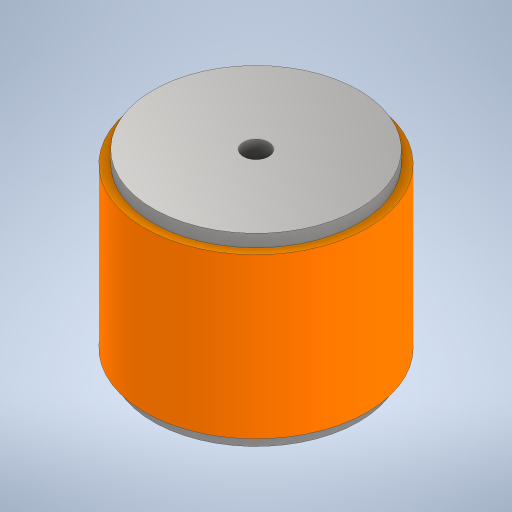
# Autodesk Inventor part: kolo
Saved by Autodesk Inventor 2024 (Build 280153000, 153)
## iProperties
Created: 2023-03-19
Part Number: kolo
Material: Všeobecné
Document SubType Name: Modeling
Designer: Simak
Density: 1 g/cm^3
Appearance: Výchozí
Author: Simak
Autodesk Inventor part; units mm, degrees
ref_plane "YZ Plane" through (0, 0, 0) normal (1, 0, 0) x (0, 1, 0)
ref_plane "XZ Plane" through (0, 0, 0) normal (0, 1, 0) x (-1, 0, 0)
ref_plane "XY Plane" through (0, 0, 0) normal (0, 0, 1) x (1, 0, 0)
sketch "Náčrt1" plane through (0, 0, 0) normal (0, 0, 1) x (1, 0, 0)
  line L0 (12.25, 0) -> (12.25, 1.5)
  line L1 (12.25, 1.5) -> (13.25, 1.5)
  line L2 (13.25, 1.5) -> (13.25, 20.5)
  line L3 (13.25, 20.5) -> (12.25, 20.5)
  line L4 (12.25, 20.5) -> (12.25, 22)
  line L5 (0, 22) -> (0, 0)
  line L6 (12.25, 22) -> (1.5, 22)
  line L7 (12.25, 0) -> (9.25, 0)
  line L8 (9.25, 0) -> (9.25, 12)
  line L9 (9.25, 12) -> (1.5, 12)
  line L10 (1.5, 12) -> (1.5, 22)
  dimension "d8" = 26.5
  dimension "d9" = 1
  dimension "d10" = 19
  dimension "d11" = 10
  dimension "d12" = 3
  dimension "d13" = 3
  dimension "d14" = 22
  dimension "d15" = 22
  constraints: 22 end point, 9 perpendicular, 2 equal length, 2 horizontal alignment, 1 coincident
  measures "d8" diameter of L2.end L5
  measures "d9" distance of L2.end L3.end
  measures "d10" distance of L1.end L2.end
  measures "d11" distance of L9.end L6.end
  measures "d12" diameter of L10 L5
  measures "d13" distance of L0.start L7.end
  measures "d14" distance of L5.start L5.end
  measures "d15" distance between parallel lines of L7 L6
revolve "Rotace1" add sketch "Náčrt1" angle 360 about axis through (0, 22, 0) along (0, -1, 0)
